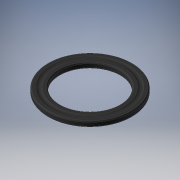
# Autodesk Inventor part: 51107 Housing washer
Saved by Autodesk Inventor 2023 (Build 270158000, 158)
## iProperties
Created: 2023-07-26
Part Number: 51107 Housing washer
Material: Generic
Catalog Web Link: www.cadenas.de
Description: With flat seet HW-
Vendor: NSK_RB
Document SubType Name: Modeling
Designer: psAdmin
Manufacturer: NSK_RB
Mass: 3.36543 g
Surface Area: 28.9991 cm^2
Volume: 3.36543 cm^3
Density: 1 g/cm^3
Appearance: PSOLRGB-175-175-175
Category: PARTsolutions
Company: NSK_RB
PSOL_IDENT_0: {$CADENAS_DATA/23d-libs/nsk_rb/roller_bearings/thrust_bearings/single_direction_tbb/with_flat_seet_h
PSOL_IDENT_1: w.prj},193 {VTYP=3D},{NB=51107 Housing washer},{LINA=51107 Housing washer},{NN=With flat seet HW},{D
PSOL_IDENT_2: ATE=27.09.2022 23:23:10},{GEOMDATE=23.08.2022 10:33:13},{VERSION=},{LINEID=6430},{WBVAR=},{WBNUMERIC=
PSOL_IDENT_3: }  {NB=51107 Housing washer},{LINA=51107 Housing washer},{KT=DUMMY},{N=18},{IDNR=},{STAN=},{NO=19},{
PSOL_IDENT_4: ORDER=51107},{SD=35},{D=52},{T=12},{T3=0.0},{T4=0},{SR=0.6},{CAN=22100},{COAN=49500},{CA=2250},{COA=
PSOL_IDENT_5: 5050},{GRE=4000},{OIL=6000},{SD1=52},{D1=37},{D2=0},{D3=0},{SB=0.0},{A=0.0},{R=0},{SDA=45},{DA=42},{
PSOL_IDENT_6: SRA=0.6},{MASS=0.081},{DIST=2.133}
NB: 51107 Housing washer
NN: With flat seet HW
NBSYN: $ORDER. Housing washer
LINA: 51107 Housing washer
CATALOG: NSK Rolling Bearing
N: 18
NO: 19
ORDER: 51107
SD: 35
D: 52
T: 12
T3: 0
T4: 0
SR: 0.6
CAN: 22100
COAN: 49500
CA: 2250
COA: 5050
GRE: 4000
OIL: 6000
SD1: 52
D1: 37
D2: 0
D3: 0
SB: 0
A: 0
R: 0
SDA: 45
DA: 42
SRA: 0.6
MASS: 0.081
SUPPLIER: NSK_RB
ARTICLENO: 51107 Housing washer
BOMINFO: 51107 Housing washer
CREATOR: CADENAS GmbH
Title: 51107 Housing washer
Author: Cadenas PARTsolutions
Autodesk Inventor part; units mm, degrees
sketch "Sketch_1" plane through (0, 0, 0) normal (0, 0, 1) x (0, 1, 0)
  line L0 (3.3333, 0) -> (0, 0)
  arc A0 (0, 19.1) -> (0.6, 18.5) centre (0.6, 19.1) ccw
  line L1 (0.6, 18.5) -> (2.7333, 18.5)
  arc A1 (2.7333, 18.5) -> (3.3333, 19.1) centre (2.7333, 19.1) ccw
  line L2 (3.3333, 19.1) -> (3.3333, 20.8756)
  arc A2 (3.3333, 23.6244) -> (3.3333, 20.8756) centre (6, 22.25) ccw
  line L3 (3.3333, 23.6244) -> (3.3333, 25.4)
  arc A3 (3.3333, 25.4) -> (2.7333, 26) centre (2.7333, 25.4) ccw
  line L4 (2.7333, 26) -> (0.6, 26)
  arc A4 (0.6, 26) -> (0, 25.4) centre (0.6, 25.4) ccw
  line L5 (0, 25.4) -> (0, 19.1)
  constraints: 12 end point, 10 point on circle, 5 centre point
revolve "Revolution1" add sketch "Sketch_1" angle 360 about axis through (0, 3.3333, 0) along (0, 1, 0)
ref_plane "HW_B_1_XY" through (-22.25, 6, 0) normal (0, 1, 0) x (0, 0, -1)
ref_plane "HW_B_1_YZ" through (-22.25, 6, 0) normal (0, 0, -1) x (-1, 0, 0)
ref_plane "HW_B_1_ZX" through (-22.25, 6, 0) normal (-1, 0, 0) x (0, 1, 0)
ref_plane "HW_B_10_XY" through (22.25, 6, 0) normal (0, 1, 0) x (0, 0, -1)
ref_plane "HW_B_10_YZ" through (22.25, 6, 0) normal (0, 0, -1) x (-1, 0, 0)
ref_plane "HW_B_10_ZX" through (22.25, 6, 0) normal (-1, 0, 0) x (0, 1, 0)
ref_plane "HW_B_11_XY" through (20.9082, 6, -7.6099) normal (0, 1, 0) x (0, 0, -1)
ref_plane "HW_B_11_YZ" through (20.9082, 6, -7.6099) normal (0, 0, -1) x (-1, 0, 0)
ref_plane "HW_B_11_ZX" through (20.9082, 6, -7.6099) normal (-1, 0, 0) x (0, 1, 0)
ref_plane "HW_B_12_XY" through (17.0445, 6, -14.302) normal (0, 1, 0) x (0, 0, -1)
ref_plane "HW_B_12_YZ" through (17.0445, 6, -14.302) normal (0, 0, -1) x (-1, 0, 0)
ref_plane "HW_B_12_ZX" through (17.0445, 6, -14.302) normal (-1, 0, 0) x (0, 1, 0)
ref_plane "HW_B_13_XY" through (11.125, 6, -19.2691) normal (0, 1, 0) x (0, 0, -1)
ref_plane "HW_B_13_YZ" through (11.125, 6, -19.2691) normal (0, 0, -1) x (-1, 0, 0)
ref_plane "HW_B_13_ZX" through (11.125, 6, -19.2691) normal (-1, 0, 0) x (0, 1, 0)
ref_plane "HW_B_14_XY" through (3.8637, 6, -21.912) normal (0, 1, 0) x (0, 0, -1)
ref_plane "HW_B_14_YZ" through (3.8637, 6, -21.912) normal (0, 0, -1) x (-1, 0, 0)
ref_plane "HW_B_14_ZX" through (3.8637, 6, -21.912) normal (-1, 0, 0) x (0, 1, 0)
ref_plane "HW_B_15_XY" through (-3.8637, 6, -21.912) normal (0, 1, 0) x (0, 0, -1)
ref_plane "HW_B_15_YZ" through (-3.8637, 6, -21.912) normal (0, 0, -1) x (-1, 0, 0)
ref_plane "HW_B_15_ZX" through (-3.8637, 6, -21.912) normal (-1, 0, 0) x (0, 1, 0)
ref_plane "HW_B_16_XY" through (-11.125, 6, -19.2691) normal (0, 1, 0) x (0, 0, -1)
ref_plane "HW_B_16_YZ" through (-11.125, 6, -19.2691) normal (0, 0, -1) x (-1, 0, 0)
ref_plane "HW_B_16_ZX" through (-11.125, 6, -19.2691) normal (-1, 0, 0) x (0, 1, 0)
ref_plane "HW_B_17_XY" through (-17.0445, 6, -14.302) normal (0, 1, 0) x (0, 0, -1)
ref_plane "HW_B_17_YZ" through (-17.0445, 6, -14.302) normal (0, 0, -1) x (-1, 0, 0)
ref_plane "HW_B_17_ZX" through (-17.0445, 6, -14.302) normal (-1, 0, 0) x (0, 1, 0)
ref_plane "HW_B_18_XY" through (-20.9082, 6, -7.6099) normal (0, 1, 0) x (0, 0, -1)
ref_plane "HW_B_18_YZ" through (-20.9082, 6, -7.6099) normal (0, 0, -1) x (-1, 0, 0)
ref_plane "HW_B_18_ZX" through (-20.9082, 6, -7.6099) normal (-1, 0, 0) x (0, 1, 0)
ref_plane "HW_B_2_XY" through (-20.9082, 6, 7.6099) normal (0, 1, 0) x (0, 0, -1)
ref_plane "HW_B_2_YZ" through (-20.9082, 6, 7.6099) normal (0, 0, -1) x (-1, 0, 0)
ref_plane "HW_B_2_ZX" through (-20.9082, 6, 7.6099) normal (-1, 0, 0) x (0, 1, 0)
ref_plane "HW_B_3_XY" through (-17.0445, 6, 14.302) normal (0, 1, 0) x (0, 0, -1)
ref_plane "HW_B_3_YZ" through (-17.0445, 6, 14.302) normal (0, 0, -1) x (-1, 0, 0)
ref_plane "HW_B_3_ZX" through (-17.0445, 6, 14.302) normal (-1, 0, 0) x (0, 1, 0)
ref_plane "HW_B_4_XY" through (-11.125, 6, 19.2691) normal (0, 1, 0) x (0, 0, -1)
ref_plane "HW_B_4_YZ" through (-11.125, 6, 19.2691) normal (0, 0, -1) x (-1, 0, 0)
ref_plane "HW_B_4_ZX" through (-11.125, 6, 19.2691) normal (-1, 0, 0) x (0, 1, 0)
ref_plane "HW_B_5_XY" through (-3.8637, 6, 21.912) normal (0, 1, 0) x (0, 0, -1)
ref_plane "HW_B_5_YZ" through (-3.8637, 6, 21.912) normal (0, 0, -1) x (-1, 0, 0)
ref_plane "HW_B_5_ZX" through (-3.8637, 6, 21.912) normal (-1, 0, 0) x (0, 1, 0)
ref_plane "HW_B_6_XY" through (3.8637, 6, 21.912) normal (0, 1, 0) x (0, 0, -1)
ref_plane "HW_B_6_YZ" through (3.8637, 6, 21.912) normal (0, 0, -1) x (-1, 0, 0)
ref_plane "HW_B_6_ZX" through (3.8637, 6, 21.912) normal (-1, 0, 0) x (0, 1, 0)
ref_plane "HW_B_7_XY" through (11.125, 6, 19.2691) normal (0, 1, 0) x (0, 0, -1)
ref_plane "HW_B_7_YZ" through (11.125, 6, 19.2691) normal (0, 0, -1) x (-1, 0, 0)
ref_plane "HW_B_7_ZX" through (11.125, 6, 19.2691) normal (-1, 0, 0) x (0, 1, 0)
ref_plane "HW_B_8_XY" through (17.0445, 6, 14.302) normal (0, 1, 0) x (0, 0, -1)
ref_plane "HW_B_8_YZ" through (17.0445, 6, 14.302) normal (0, 0, -1) x (-1, 0, 0)
ref_plane "HW_B_8_ZX" through (17.0445, 6, 14.302) normal (-1, 0, 0) x (0, 1, 0)
ref_plane "HW_B_9_XY" through (20.9082, 6, 7.6099) normal (0, 1, 0) x (0, 0, -1)
ref_plane "HW_B_9_YZ" through (20.9082, 6, 7.6099) normal (0, 0, -1) x (-1, 0, 0)
ref_plane "HW_B_9_ZX" through (20.9082, 6, 7.6099) normal (-1, 0, 0) x (0, 1, 0)
ref_plane "HW_SW_XY" through (0, 0, 0) normal (0, 1, 0) x (0, 0, -1)
ref_plane "HW_SW_YZ" through (0, 0, 0) normal (0, 0, -1) x (-1, 0, 0)
ref_plane "HW_SW_ZX" through (0, 0, 0) normal (-1, 0, 0) x (0, 1, 0)
body "Solid1"
